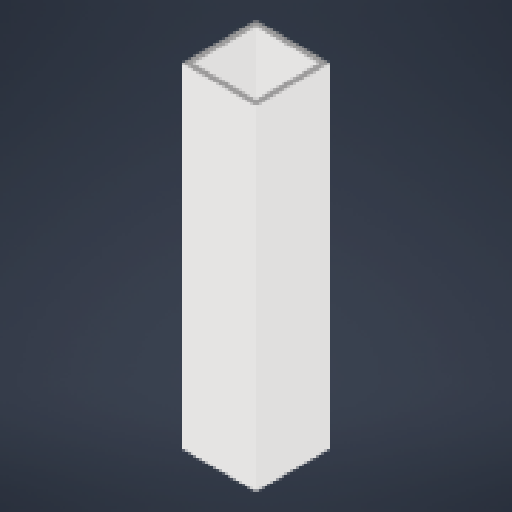
# Autodesk Inventor part: shock_absorber_holder
Saved by Autodesk Inventor 2024 (Build 280153000, 153)
## iProperties
Created: 2023-04-29
Part Number: shock_absorber_holder
Material: Типовые
Document SubType Name: Modeling
Designer: user
Density: 1 g/cm^3
Appearance: По умолчанию
Author: user
Autodesk Inventor part; units mm, degrees
ref_plane "YZ Plane" through (0, 0, 0) normal (1, 0, 0) x (0, 1, 0)
ref_plane "XZ Plane" through (0, 0, 0) normal (0, 1, 0) x (-1, 0, 0)
ref_plane "XY Plane" through (0, 0, 0) normal (0, 0, 1) x (1, 0, 0)
sketch "Эскиз1" plane through (0, 0, 0) normal (0, 0, 1) x (1, 0, 0)
  line L0 (0, -20) -> (90, -20) construction
  line L1 (0, 0) -> (90, 0) construction
  line L2 (35, -20) -> (35, 392) construction
  line L3 (35, 0) -> (15, 0)
  line L4 (15, 0) -> (15, -20)
  line L5 (15, -20) -> (35, -20)
  line L6 (35, -20) -> (35, 0)
  line L7 (33.5, -1.5) -> (16.5, -1.5)
  line L8 (16.5, -1.5) -> (16.5, -18.5)
  line L9 (16.5, -18.5) -> (33.5, -18.5)
  line L10 (33.5, -18.5) -> (33.5, -1.5)
  point P0 (25, -18.5)
  point P1 (25, -20)
  point P2 (33.5, -10)
  point P3 (35, -10)
  dimension "d0" = 20
  dimension "d1" = 1.5
  constraints: 16 end point, 4 midpoint, 4 parallel, 3 perpendicular, 3 point on line, 2 horizontal, 1 horizontal alignment, 1 vertical alignment
  measures "d0" distance of L4.end L2.start
  measures "d1" horizontal distance of L4.end L8.end
extrude "Выдавливание1" add sketch "Эскиз1" along normal blind 90
